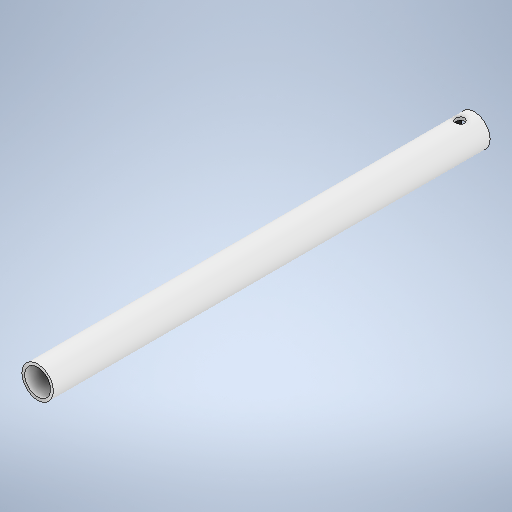
# Autodesk Inventor part: Shifter PVC
Saved by Autodesk Inventor 2025.2 (Build 292293000, 293)
## iProperties
Created: 2025-02-09
Part Number: Shifter PVC
Material: PVC-Piping
Document SubType Name: Modeling
Designer: eason
Density: 1.4 g/cm^3
Appearance: Smooth - White
Author: eason
Autodesk Inventor part; units mm, degrees
ref_plane "YZ Plane" through (0, 0, 0) normal (1, 0, 0) x (0, 1, 0)
ref_plane "XY Plane" through (0, 0, 0) normal (0, 0, 1) x (1, 0, 0)
sketch "Sketch1" plane through (0, 0, 0) normal (0, 0, 1) x (1, 0, 0)
  circle A0 centre (0, 0) radius 10.75
  circle A1 centre (0, 0) radius 8.85
  dimension "d0" = 21.5
  dimension "d1" = 17.7
  constraints: 2 centre point, 2 coincident
  measures "d0" diameter of A0
  measures "d1" diameter of A1
extrude "Extrusion1" add sketch "Sketch1" along normal blind 300
ref_plane "Work Plane1" through (0, -10.75, 0) normal (0, 1, 0) x (-1, 0, 0)
sketch "Sketch2" plane through (0, -10.75, 0) normal (0, 1, 0) x (-1, 0, 0)
  circle A0 centre (0, 10) radius 3
  line L0 (0, -60) -> (0, 360) projected
  point P0 (0, 0)
  dimension "d4" = 6
  dimension "d5" = 10
  constraints: 1 centre point, 1 point on line
  measures "d4" diameter of A0
  measures "d5" distance of point (0, 0) A0.centre
extrude "Extrusion2" cut sketch "Sketch2" along normal through all
body "Solid1"
